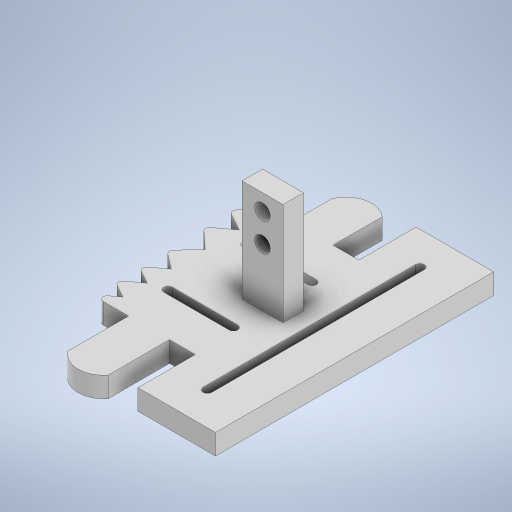
# Autodesk Inventor part: camera_cutout
Saved by Autodesk Inventor 2024 (Build 280153000, 153)
## iProperties
Created: 2023-12-03
Part Number: camera_cutout
Material: Generic
Document SubType Name: Modeling
Designer: dimademler
Density: 1 g/cm^3
Appearance: Default
Author: dimademler
Autodesk Inventor part; units mm, degrees
ref_plane "YZ Plane" through (0, 0, 0) normal (1, 0, 0) x (0, 1, 0)
ref_plane "XZ Plane" through (0, 0, 0) normal (0, 1, 0) x (-1, 0, 0)
ref_plane "XY Plane" through (0, 0, 0) normal (0, 0, 1) x (1, 0, 0)
sketch "Sketch1" plane through (0, 0, 0) normal (0, 0, 1) x (1, 0, 0)
  line L0 (0, 0) -> (0, 38.1)
  line L1 (0, 38.1) -> (-12.7, 38.1)
  line L2 (-12.7, 38.1) -> (-12.7, 0)
  line L3 (-12.7, 0) -> (0, 0)
  dimension "d0" = 38.1
  dimension "d1" = 12.7
  constraints: 8 end point, 2 parallel, 1 perpendicular, 1 vertical
  measures "d0" distance of L0.start L0.end
  measures "d1" distance of L1.end L0.end
extrude "Extrusion1" add sketch "Sketch1" along normal blind 6.35
sketch "Sketch2" plane through (0, 0, 6.35) normal (0, 0, 1) x (1, 0, 0)
  line L0 (0, 38.1) -> (-12.7, 38.1) projected
  line L1 (-12.7, 38.1) -> (-12.7, 0) projected
  line L2 (-12.7, 0) -> (0, 0) projected
  line L3 (0, 0) -> (0, 38.1) projected
  line L4 (-6.35, 38.1) -> (-6.35, 0) construction
  line L5 (-6.35, 38.1) -> (-6.35, 33.02)
  circle A0 centre (-6.35, 33.02) radius 2.413
  line L6 (-6.35, 33.02) -> (-6.35, 24.257)
  circle A1 centre (-6.35, 24.257) radius 2.413
  dimension "d4" = 5.08
  dimension "d5" = 4.826
  dimension "d6" = 8.763
  dimension "d7" = 4.826
  constraints: 6 end point, 2 centre point, 2 coincident, 2 midpoint, 2 point on line
  measures "d4" distance of L4.start L5.end
  measures "d5" diameter of A0
  measures "d6" distance of L6.start L6.end
  measures "d7" diameter of A1
extrude "Extrusion2" cut sketch "Sketch2" against normal up to next contours A1 | A0 L6 L5 | L5 L6 A0
sketch "Sketch3" plane through (-12.7, 0, 0) normal (0, -1, 0) x (1, 0, 0)
  line L0 (0, 0) -> (12.7, 0) projected
  line L1 (12.7, 0) -> (12.7, 6.35) projected
  line L2 (0, 6.35) -> (12.7, 6.35) projected
  line L3 (0, 0) -> (0, 6.35) projected
  line L4 (0, 3.175) -> (12.7, 3.175) construction
  line L5 (6.35, 6.35) -> (6.35, 0) construction
  line L6 (-19.05, -22.225) -> (-19.05, 28.575)
  line L7 (-19.05, 28.575) -> (31.75, 28.575)
  line L8 (31.75, 28.575) -> (31.75, -22.225)
  line L9 (31.75, -22.225) -> (-19.05, -22.225)
  line L10 (-19.05, -22.225) -> (31.75, 28.575) construction
  line L11 (-19.05, 28.575) -> (31.75, -22.225) construction
  point P0 (6.35, 3.175)
  dimension "d10" = 50.8
  dimension "d11" = 50.8
  constraints: 16 end point, 7 midpoint, 2 parallel, 1 perpendicular, 1 vertical
  measures "d10" distance of L6.start L6.end
  measures "d11" distance of L6.end L7.end
extrude "Extrusion3" add sketch "Sketch3" against normal blind 6.35
sketch "Sketch4" plane through (-31.75, 0, 28.575) normal (0, -1, 0) x (1, 0, 0)
  line L0 (50.8, -50.8) -> (50.8, 0) projected
  line L1 (50.8, 0) -> (0, 0) projected
  line L2 (0, 0) -> (0, -50.8) projected
  line L3 (0, -50.8) -> (50.8, -50.8) projected
  line L4 (0, -25.4) -> (50.8, -25.4) construction
  line L5 (0, -25.4) -> (0, -13.208)
  line L6 (0, -13.208) -> (5.08, -13.208)
  line L7 (5.08, -13.208) -> (25.4, -13.208) construction
  line L8 (5.08, -14.5288) -> (25.4, -14.5288)
  line L9 (25.4, -11.8872) -> (5.08, -11.8872)
  arc A0 (5.08, -11.8872) -> (5.08, -14.5288) centre (5.08, -13.208) ccw
  arc A1 (25.4, -14.5288) -> (25.4, -11.8872) centre (25.4, -13.208) ccw
  line L10 (5.08, -36.2712) -> (25.4, -36.2712)
  line L11 (25.4, -38.9128) -> (5.08, -38.9128)
  arc A2 (5.08, -36.2712) -> (5.08, -38.9128) centre (5.08, -37.592) ccw
  arc A3 (25.4, -38.9128) -> (25.4, -36.2712) centre (25.4, -37.592) ccw
  point P0 (31.75, -28.575)
  point P1 (15.24, -13.208)
  dimension "d14" = 12.192
  dimension "d16" = 5.08
  dimension "d17" = 20.32
  dimension "d18" = 2.6416
  constraints: 18 end point, 8 point on circle, 6 symmetric about line, 4 centre point, 4 tangent, 3 midpoint, 2 horizontal, 1 parallel, 1 point on line, 2 other
  measures "d14" distance of L4.start L5.end
  measures "d16" distance of L5.end L6.end
  measures "d17" distance of L6.end L7.end
  measures "d18" diameter of A1
extrude "Extrusion4" cut sketch "Sketch4" against normal blind 6.35 contours A0 L9 A1 L8 | L10 A3 L11 A2
sketch "Sketch6" plane through (-31.75, 0, 28.575) normal (0, -1, 0) x (1, 0, 0)
  line L0 (25.4, -14.5288) -> (5.08, -14.5288) projected
  arc A0 (5.08, -11.8872) -> (5.08, -14.5288) centre (5.08, -13.208) ccw projected
  line L1 (5.08, -11.8872) -> (25.4, -11.8872) projected
  arc A1 (25.4, -14.5288) -> (25.4, -11.8872) centre (25.4, -13.208) ccw projected
  arc A2 (5.08, -36.2712) -> (5.08, -38.9128) centre (5.08, -37.592) ccw projected
  line L2 (5.08, -36.2712) -> (25.4, -36.2712) projected
  arc A3 (25.4, -38.9128) -> (25.4, -36.2712) centre (25.4, -37.592) ccw projected
  line L3 (25.4, -38.9128) -> (5.08, -38.9128) projected
  line L4 (50.8, -50.8) -> (50.8, 0) projected
  line L5 (50.8, 0) -> (0, 0) projected
  line L6 (0, 0) -> (0, -50.8) projected
  line L7 (0, -50.8) -> (50.8, -50.8) projected
  line L8 (26.7208, -13.208) -> (26.7208, -50.8)
  line L9 (26.7208, -13.208) -> (26.7208, 0)
  line L10 (26.7208, 0) -> (26.7208, 17.78)
  line L11 (26.7208, -50.8) -> (26.7208, -68.58)
  line L12 (26.7208, 17.78) -> (50.8, 17.78)
  line L13 (50.8, 17.78) -> (50.8, 0)
  line L14 (26.7208, -68.58) -> (50.8, -68.58)
  line L15 (50.8, -68.58) -> (50.8, -50.8)
  point P0 (31.75, -28.575)
  dimension "d23" = 17.78
  dimension "d24" = 17.78
  constraints: 16 end point, 5 perpendicular, 4 point on line, 1 horizontal, 1 point on circle, 1 vertical
  measures "d23" distance of L9.end L10.end
  measures "d24" distance of L8.end L11.end
extrude "Extrusion5" add sketch "Sketch6" against normal blind 6.35 contours L10 L12 L13 L5 | L7 L15 L14 L11
sketch "Sketch7" plane through (-31.75, 0, -22.225) normal (0, -1, 0) x (1, 0, 0)
  line L0 (25.4, 36.2712) -> (5.08, 36.2712) projected
  arc A0 (5.08, 38.9128) -> (5.08, 36.2712) centre (5.08, 37.592) ccw projected
  line L1 (5.08, 38.9128) -> (25.4, 38.9128) projected
  arc A1 (25.4, 36.2712) -> (25.4, 38.9128) centre (25.4, 37.592) ccw projected
  arc A2 (5.08, 14.5288) -> (5.08, 11.8872) centre (5.08, 13.208) ccw projected
  line L2 (5.08, 14.5288) -> (25.4, 14.5288) projected
  arc A3 (25.4, 11.8872) -> (25.4, 14.5288) centre (25.4, 13.208) ccw projected
  line L3 (25.4, 11.8872) -> (5.08, 11.8872) projected
  line L4 (50.8, -17.78) -> (50.8, 68.58) projected
  line L5 (50.8, 68.58) -> (26.7208, 68.58) projected
  line L6 (26.7208, 68.58) -> (26.7208, 50.8) projected
  line L7 (26.7208, 50.8) -> (0, 50.8) projected
  line L8 (0, 50.8) -> (0, 0) projected
  line L9 (0, 0) -> (26.7208, 0) projected
  line L10 (26.7208, 0) -> (26.7208, -17.78) projected
  line L11 (26.7208, -17.78) -> (50.8, -17.78) projected
  line L12 (25.4, 37.592) -> (25.4, 13.208) construction
  line L13 (25.4, 25.4) -> (50.8, 25.4) construction
  line L14 (38.1, -7.62) -> (38.1, 58.42) construction
  line L15 (39.4335, -7.62) -> (39.4335, 58.42)
  line L16 (36.7665, 58.42) -> (36.7665, -7.62)
  arc A4 (36.7665, -7.62) -> (39.4335, -7.62) centre (38.1, -7.62) ccw
  arc A5 (39.4335, 58.42) -> (36.7665, 58.42) centre (38.1, 58.42) ccw
  point P0 (31.75, 22.225)
  point P1 (38.1, 25.4)
  dimension "d27" = 33.02
  dimension "d28" = 2.667
  constraints: 12 end point, 4 midpoint, 4 point on circle, 4 tangent, 2 centre point, 1 parallel, 1 perpendicular, 1 vertical
  measures "d27" distance of point (38.1, 25.4) L14.end
  measures "d28" diameter of A5
extrude "Extrusion6" cut sketch "Sketch7" against normal blind 6.35 contours A4 L16 A5 L15
sketch "Sketch8" plane through (-31.75, 0, -22.225) normal (0, -1, 0) x (1, 0, 0)
  line L0 (0, 0) -> (0, 50.8) projected
  line L1 (0, 0) -> (-6.9749, 6.5838)
  line L2 (-6.9749, 6.5838) -> (0, 10.4686)
  line L3 (0, 10.4686) -> (-6.3127, 15.1611)
  line L4 (-6.3127, 15.1611) -> (0, 20.9868)
  line L5 (-5.6991, 27.1623) -> (0, 31.5381)
  line L6 (0, 20.9868) -> (-5.6991, 27.1623)
  line L7 (0, 31.5381) -> (-5.7764, 35.832)
  line L8 (-5.7764, 35.832) -> (0, 39.0492)
  line L9 (-5.4281, 43.0842) -> (0, 39.0492)
  line L10 (-5.7764, 43.343) -> (0, 46.5602)
  line L11 (-5.7036, 50.8) -> (0, 50.8)
  line L12 (0, 50.8) -> (0, 46.5602)
  line L13 (-5.7036, 50.8) -> (0, 46.5602)
  line L14 (-5.7764, 43.343) -> (0, 39.0492)
  point P0 (31.75, 22.225)
  point P1 (-5.4281, 43.0842)
  constraints: 28 end point, 6 point on line, 5 parallel, 2 perpendicular, 1 collinear, 1 horizontal
extrude "Extrusion7" add sketch "Sketch8" against normal blind 6.35
fillet "Fillet1" radius 1.27 1 edges at (-38.7249, 3.175, -15.6412)
fillet "Fillet2" radius 1.27 1 edges at (-38.0627, 3.175, -7.0639)
fillet "Fillet3" radius 1.27 4 edges at (-37.4491, 3.175, 4.9373) (-37.5264, 3.175, 13.607) (-37.5264, 3.175, 21.118) (-37.4536, 3.175, 28.575)
sketch "Sketch9" plane through (-5.0292, 0, -40.005) normal (0, -1, 0) x (1, 0, 0)
  line L0 (-26.7208, 17.78) -> (0, 17.78) projected
  line L1 (-7.995, 17.78) -> (-7.995, 5.2737)
  line L2 (-20.7092, 17.78) -> (-20.7092, 5.4549)
  arc A0 (-20.7092, 5.4549) -> (-7.995, 2.5659) centre (-13.3604, 8.3747) ccw
  line L3 (-7.995, 5.2737) -> (-7.995, 2.5659)
  line L4 (24.0792, 0) -> (24.0792, 86.36) projected
  line L5 (24.0792, 43.18) -> (-30.9425, 43.18) construction
  line L6 (-28.5871, 68.58) -> (0, 68.58) projected
  line L7 (-7.995, 68.58) -> (-7.995, 82.6845)
  line L8 (-20.7092, 68.58) -> (-20.7092, 82.6845)
  line L9 (-20.7092, 82.6845) -> (-20.7092, 87.4507)
  line L10 (-7.995, 82.6845) -> (-7.995, 87.6044)
  arc A1 (-7.995, 87.6044) -> (-20.7092, 87.4507) centre (-14.2936, 82.6845) ccw
  point P0 (5.0292, 40.005)
  constraints: 16 end point, 7 vertical, 4 point on circle, 4 point on line, 2 centre point, 1 horizontal, 1 midpoint
extrude "Extrusion8" add sketch "Sketch9" against normal blind 6.35
body "Solid1"
